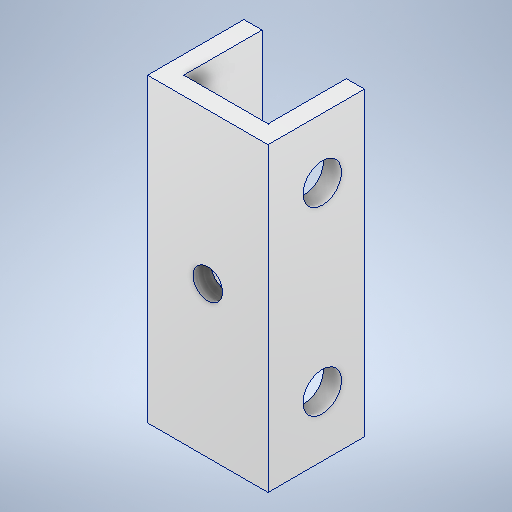
# Autodesk Inventor part: x_belt_anchor
Saved by Autodesk Inventor 2025 (Build 290162000, 162)
## iProperties
Created: 2024-04-25
Part Number: x_belt_anchor
Material: Hliník 6061
Document SubType Name: Modeling
Designer: rader
Density: 2.7 g/cm^3
Appearance: Hliník – plochý
Author: rader
Autodesk Inventor part; units mm, degrees
ref_plane "YZ Plane" through (0, 0, 0) normal (1, 0, 0) x (0, 1, 0)
ref_plane "XZ Plane" through (0, 0, 0) normal (0, 1, 0) x (-1, 0, 0)
ref_plane "XY Plane" through (0, 0, 0) normal (0, 0, 1) x (1, 0, 0)
sketch "Náčrt1" plane through (0, 0, 0) normal (0, 0, 1) x (1, 0, 0)
  line L0 (-5, 8) -> (-5, 0)
  line L1 (-5, 0) -> (5, 0)
  line L2 (5, 0) -> (5, 8)
  line L3 (5, 8) -> (3.5, 8)
  line L4 (3.5, 8) -> (3.5, 1.5)
  line L5 (3.5, 1.5) -> (-3.5, 1.5)
  line L6 (-3.5, 1.5) -> (-3.5, 8)
  line L7 (-3.5, 8) -> (-5, 8)
  line L8 (-7, 0) -> (7, 0) projected
  line L9 (0, 9.6) -> (0, -1.6) projected
  point P0 (0, 0)
  dimension "d0" = 8
  dimension "d1" = 10
  dimension "d2" = 1.5
  dimension "d3" = 1.5
  dimension "d4" = 1.5
  constraints: 16 end point, 6 perpendicular, 1 collinear, 1 parallel, 1 point on line, 1 vertical, 1 other
  measures "d0" distance of L1.end L2.end
  measures "d1" distance of L0.end L1.end
  measures "d2" distance between parallel lines of L4 L2
  measures "d3" distance between parallel lines of L5 L1
  measures "d4" distance between parallel lines of L0 L6
extrude "Vysunutí1" add sketch "Náčrt1" along normal mid plane 25
sketch "Náčrt2" plane through (5, 0, 12.5) normal (1, 0, 0) x (0, 0, -1)
  line L0 (25, 8) -> (25, 0) projected
  line L1 (0, 0) -> (0, 8) projected
  line L2 (25, 8) -> (0, 8) projected
  point P0 (12.5, 0)
  point P1 (5, 4.5)
  point P2 (20, 4.5)
  dimension "d7" = 5
  dimension "d8" = 5
  dimension "d9" = 3.5
  dimension "d10" = 3.5
  measures "d7" distance from line of L0 point (20, 4.5)
  measures "d8" distance from line of L1 point (5, 4.5)
  measures "d9" distance from line of L2 point (20, 4.5)
  measures "d10" distance from line of L2 point (5, 4.5)
hole "Díra1" at (5, 4.5, 7.5) at (5, 4.5, -7.5) direction (-1, 0, 0) diameter 2.459 end through all counterbore diameter 3.2 counterbore depth 2 thread size "M3x0.5" class "6H" standard "ISO Metric profile"
sketch "Náčrt3" plane through (-3.5, 1.5, 12.5) normal (0, 1, 0) x (1, 0, 0)
  line L0 (0, 25) -> (0, 0) projected
  point P0 (3.5, 12.5)
  point P1 (3.5, 12.5)
  constraints: 1 coincident
hole "Díra2" at (0, 1.5, 0) direction (0, -1, 0) diameter 2.459 end through all thread size "M3x0.5" class "6H" standard "ISO Metric profile"
